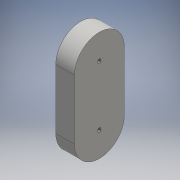
# Autodesk Inventor part: gasienice
Saved by Autodesk Inventor 2016 (Build 200138000, 138)
## iProperties
Created: 2015-11-09
Part Number: gasienice
Material: Ogólny
Document SubType Name: Modeling
Designer: Mrianura
Density: 1 g/cm^3
Appearance: Domyślna
Author: Mrianura
Autodesk Inventor part; units mm, degrees
ref_plane "YZ Plane" through (0, 0, 0) normal (1, 0, 0) x (0, 1, 0)
ref_plane "XZ Plane" through (0, 0, 0) normal (0, 1, 0) x (-1, 0, 0)
ref_plane "XY Plane" through (0, 0, 0) normal (0, 0, 1) x (1, 0, 0)
sketch "Szkic1" plane through (0, 0, 0) normal (1, 0, 0) x (0, 1, 0)
  line L0 (0, -24) -> (0, 24)
  circle A0 centre (20, 24) radius 20
  circle A1 centre (20, -24) radius 20
  line L1 (40, 24) -> (40, -24)
  line L2 (0, -24) -> (0, 24)
  point P0 (0, 0)
  dimension "d0" = 24
  dimension "d1" = 48
  dimension "d2" = 40
  constraints: 6 end point, 3 vertical, 2 horizontal alignment, 1 collinear, 4 other
  measures "d0" distance of point (0, 0) L0.start
  measures "d1" distance of L0.start L0.end
  measures "d2" distance of L0.end L1.start
extrude "Wyciągnięcie proste1" add sketch "Szkic1" along normal blind 15 contours A1 | A0
sketch "Szkic2" plane through (15, 20, -24) normal (1, 0, 0) x (0, 0, -1)
  circle A0 centre (0, 0) radius 20 projected
  line L0 (0, -20) -> (-48, -20)
  circle A1 centre (-48, 0) radius 20 projected
  line L1 (0, 20) -> (-48, 20)
  line L2 (-48, 20) -> (-48, -20)
  line L3 (0, 20) -> (0, -20)
  point P0 (-24, -20)
  constraints: 8 end point, 5 point on circle, 2 tangent, 1 parallel, 1 point on line
extrude "Wyciągnięcie proste2" add sketch "Szkic2" against normal blind 15 contours A0 L0 A1 L1
sketch "Szkic3" plane through (15, 0, 0) normal (1, 0, 0) x (0, 0, -1)
  line L0 (0, 0) -> (0, 20)
  line L1 (-24, 40) -> (24, 40) projected
  line L2 (0, 20) -> (24, 20)
  line L3 (24, 20) -> (-24, 20)
  arc A0 (22.882, 21) -> (25.118, 21) centre (24, 20) ccw
  arc A1 (-25.118, 21) -> (-22.882, 21) centre (-24, 20) ccw
  line L4 (-24, 18.5) -> (-24, 21)
  line L5 (-24, 21) -> (-22.882, 21)
  line L6 (-24, 21) -> (-25.118, 21)
  line L7 (24, 18.5) -> (24, 21)
  line L8 (24, 21) -> (25.118, 21)
  line L9 (24, 21) -> (22.882, 21)
  dimension "d7" = 20
  dimension "d8" = 24
  dimension "d9" = 48
  dimension "d10" = 3
  dimension "d11" = 3
  dimension "d12" = 2.5
  dimension "d13" = 2.5
  constraints: 18 end point, 6 point on circle, 5 point on line, 3 perpendicular, 2 centre point, 2 coincident, 1 vertical
  measures "d7" distance of L0.start L0.end
  measures "d8" distance of L0.end L2.end
  measures "d9" distance of L2.end L3.end
  measures "d10" diameter of A0
  measures "d11" diameter of A1
  measures "d12" distance of L4.start L4.end
  measures "d13" distance of L7.start L7.end
hole "Otwór1" at (15, 20, 24) direction (-1, 0, 0) diameter 3 end through all
sketch "Szkic4" plane through (15, 0, 0) normal (1, 0, 0) x (0, 0, -1)
  circle A0 centre (-24, 20) radius 1.5 projected
  line L0 (-24, 20) -> (24, 20)
  point P0 (0, 0)
  dimension "d21" = 48
  constraints: 2 end point, 1 horizontal
  measures "d21" distance of L0.start L0.end
hole "Otwór2" at (15, 20, -24) direction (-1, 0, 0) diameter 3 end through all
sketch "Szkic5" plane through (15, 0, 0) normal (1, 0, 0) x (0, 0, -1)
  circle A0 centre (-24, 20) radius 1.5 projected
  line L0 (-24, 18.5) -> (-24, 21)
  line L1 (-24, 21) -> (-22.882, 21)
  line L2 (-24, 21) -> (-25.118, 21)
  circle A1 centre (24, 20) radius 1.5 projected
  line L3 (24, 18.5) -> (24, 21)
  line L4 (24, 21) -> (25.118, 21)
  line L5 (24, 21) -> (22.882, 21)
  point P0 (0, 0)
  dimension "d29" = 2.5
  dimension "d30" = 2.5
  constraints: 12 end point, 6 point on circle, 3 point on line, 1 horizontal, 1 perpendicular, 1 vertical
  measures "d29" distance of L0.start L0.end
  measures "d30" distance of L3.start L3.end
extrude "Wyciągnięcie proste3" add sketch "Szkic5" against normal blind 15 contours L1 L2 A0 | L4 L5 A1
